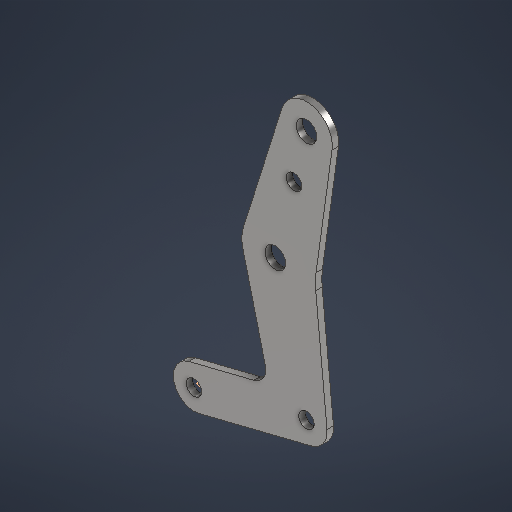
# Autodesk Inventor part: Base
Saved by Autodesk Inventor 2025.4 (Build 294407000, 407)
## iProperties
Created: 2026-05-26
Part Number: Base
Material: Steel, Mild
Document SubType Name: Modeling
Designer: VuQuan
Density: 7.85 g/cm^3
Appearance: Semi-Polished
Author: VuQuan
Autodesk Inventor part; units mm, degrees
ref_plane "YZ Plane" through (0, 0, 0) normal (1, 0, 0) x (0, 1, 0)
ref_plane "XZ Plane" through (0, 0, 0) normal (0, 1, 0) x (-1, 0, 0)
ref_plane "XY Plane" through (0, 0, 0) normal (0, 0, 1) x (1, 0, 0)
sketch "Sketch1" plane through (0, 0, 0) normal (0, 0, 1) x (1, 0, 0)
  line L0 (45.5987, 3.1241) -> (1.9354, -7.7624)
  arc A0 (-1.9354, 7.7624) -> (1.9354, -7.7624) centre (0, 0) ccw
  line L1 (-1.9354, 7.7624) -> (23.2923, 14.0523)
  line L2 (27.6626, 21.3256) -> (18.9534, 56.2563)
  line L3 (19.1648, 63.2974) -> (34.123, 110.9131)
  arc A1 (53.5672, 106.5326) -> (34.123, 110.9131) centre (43.6633, 107.9161) ccw
  line L4 (53.5672, 106.5326) -> (47.3852, 62.2768)
  line L5 (47.2596, 56.1398) -> (51.625, 11.668)
  arc A2 (45.5987, 3.1241) -> (51.625, 11.668) centre (43.6633, 10.8865) ccw
  circle A3 centre (0, 0) radius 3
  circle A4 centre (43.6633, 10.8865) radius 3
  arc A5 (23.2923, 14.0523) -> (27.6626, 21.3256) centre (21.8408, 19.8741) ccw
  arc A6 (19.1648, 63.2974) -> (18.9534, 56.2563) centre (31.5672, 59.4013) ccw
  circle A7 centre (31.5672, 59.4013) radius 4
  line L6 (43.6633, 107.9161) -> (43.6633, 10.8865) construction
  line L7 (31.5672, 59.4013) -> (43.6633, 10.8865) construction
  line L8 (43.6633, 10.8865) -> (0, 0) construction
  line L9 (31.5672, 59.4013) -> (43.6633, 107.9161) construction
  arc A8 (47.3852, 62.2768) -> (47.2596, 56.1398) centre (73.1352, 58.6798) ccw
  circle A9 centre (43.6633, 107.9161) radius 4
  circle A10 centre (38.8249, 88.5101) radius 3
  dimension "d0" = 6
  dimension "d1" = 8
  dimension "d2" = 45
  dimension "d3" = 6
  dimension "d4" = 6
  dimension "d5" = 13
  dimension "d6" = 8
  dimension "d7" = 50
  dimension "d8" = 50
  dimension "d9" = 10
  dimension "d10" = 26
  dimension "d11" = 14
  dimension "d12" = 8
  dimension "d13" = 6
  dimension "d14" = 20
  constraints: 20 end point, 12 point on circle, 12 tangent, 11 centre point, 5 coincident, 2 parallel, 2 perpendicular, 1 equal length, 1 equal radius, 1 point on line, 1 vertical
  measures "d0" diameter of A3
  measures "d1" radius of A0
  measures "d2" distance of A0.centre A2.centre
  measures "d3" diameter of A4
  measures "d4" radius of A5
  measures "d5" radius of A6
  measures "d6" diameter of A7
  measures "d7" distance of A2.centre A6.centre
  measures "d8" distance of L7.start L6.start
  measures "d9" radius of A1
  measures "d10" radius of A8
  measures "d11" angle of L6 L9
  measures "d12" diameter of A9
  measures "d13" diameter of A10
  measures "d14" distance of L6.start A10.centre
extrude "Extrusion1" add sketch "Sketch1" along normal blind 2.5
body "Solid1"
